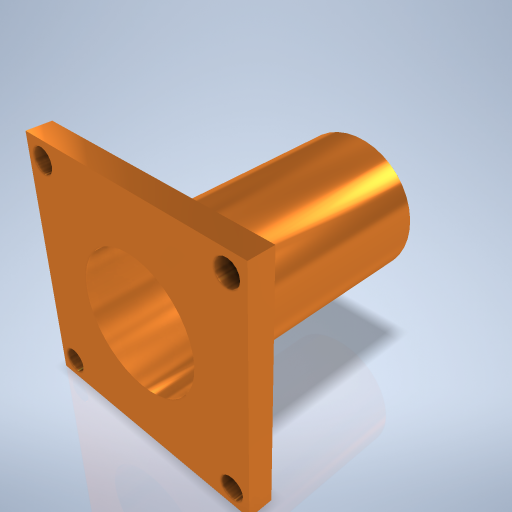
# Autodesk Inventor part: candle_cylinder
Saved by Autodesk Inventor 2024.2 (Build 282272000, 272)
## iProperties
Created: 2024-05-14
Part Number: candle_cylinder
Material: Gold
Document SubType Name: Modeling
Designer: Fabri
Density: 19.3 g/cm^3
Appearance: Metall - 1600F (heiß)
Author: Fabri
Autodesk Inventor part; units mm, degrees
ref_plane "YZ Plane" through (0, 0, 0) normal (1, 0, 0) x (0, 1, 0)
ref_plane "XZ Plane" through (0, 0, 0) normal (0, 1, 0) x (-1, 0, 0)
ref_plane "XY Plane" through (0, 0, 0) normal (0, 0, 1) x (1, 0, 0)
sketch "Skizze1" plane through (0, 0, 0) normal (0, 1, 0) x (-1, 0, 0)
  circle A0 centre (0, 0) radius 14
  dimension "d0" = 28
  constraints: 1 centre point, 1 coincident
  measures "d0" diameter of A0
extrude "Extrusion1" add sketch "Skizze1" along normal blind 51
sketch "Skizze2" plane through (0, 0, 0) normal (0, -1, 0) x (1, 0, 0)
  line L0 (-25, 25) -> (25, 25)
  line L1 (25, 25) -> (25, -25)
  line L2 (25, -25) -> (-25, -25)
  line L3 (-25, -25) -> (-25, 25)
  line L4 (-25, 25) -> (25, -25) construction
  line L5 (25, 25) -> (-25, -25) construction
  point P0 (0, 0)
  dimension "d3" = 50
  dimension "d4" = 50
  constraints: 12 end point, 2 midpoint, 2 parallel, 1 horizontal, 1 perpendicular
  measures "d3" distance of L1.end L2.end
  measures "d4" distance of L0.end L1.end
extrude "Extrusion2" add sketch "Skizze2" along normal mid plane 5
chamfer "Fasen1" distance 1 angle 45 1 edges at (14, 51, 0)
sketch "Skizze3" plane through (0, -2.5, 0) normal (0, -1, 0) x (1, 0, 0)
  point P0 (0, 0)
  point P1 (0, 0)
  constraints: 1 coincident
hole "Bohrung1" at (0, -2.5, 0) direction (0, 1, 0) diameter 27 end through all
sketch "Skizze4" plane through (0, -2.5, 0) normal (0, -1, 0) x (1, 0, 0)
  line L0 (-25, -25) -> (-25, 25) projected
  line L1 (-25, 0) -> (25, 0) construction
  line L2 (25, 25) -> (25, -25) projected
  line L3 (-25, 25) -> (25, 25) projected
  line L4 (0, 25) -> (0, -21.9496) construction
  point P0 (0, 0)
  point P1 (-21.124, -21.124)
  point P2 (-21.124, 21.124)
  point P3 (21.124, -21.124)
  point P4 (21.124, 21.124)
  dimension "d30" = 42.248
  dimension "d31" = 42.248
  dimension "d32" = 42.248
  dimension "d33" = 42.248
  constraints: 4 end point, 3 midpoint, 2 horizontal alignment, 2 symmetric about line, 2 vertical alignment, 1 vertical
  measures "d30" distance of point (21.124, 21.124) point (-21.124, 21.124)
  measures "d31" distance of point (-21.124, -21.124) point (-21.124, 21.124)
  measures "d32" distance of point (21.124, -21.124) point (21.124, 21.124)
  measures "d33" distance of point (21.124, -21.124) point (-21.124, -21.124)
hole "Bohrung2" at (-21.124, -2.5, -21.124) at (-21.124, -2.5, 21.124) at (21.124, -2.5, -21.124) at (21.124, -2.5, 21.124) direction (0, 1, 0) diameter 5 depth 5
